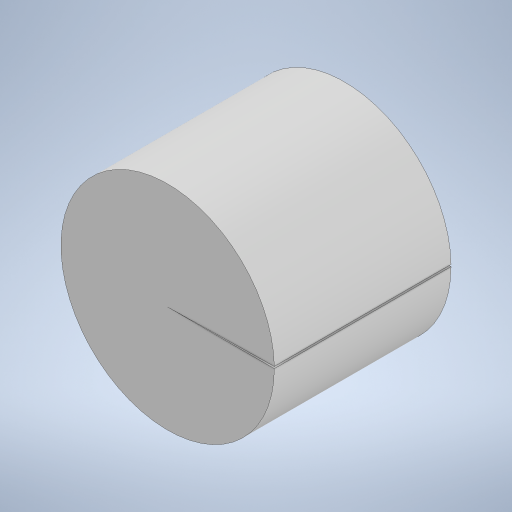
# Autodesk Inventor part: Espira_01_desarrollo
Saved by Autodesk Inventor 2024 (Build 280153000, 153)
## iProperties
Created: 2026-01-07
Part Number: Espira_01_desarrollo
Material: Generic
Document SubType Name: Modeling
Designer: eduso
Density: 1 g/cm^3
Appearance: Default
Author: eduso
Autodesk Inventor part; units mm, degrees
ref_plane "YZ Plane" through (0, 0, 0) normal (1, 0, 0) x (0, 1, 0)
ref_plane "XZ Plane" through (0, 0, 0) normal (0, 1, 0) x (-1, 0, 0)
ref_plane "XY Plane" through (0, 0, 0) normal (0, 0, 1) x (1, 0, 0)
sketch "Sketch1" plane through (0, 0, 0) normal (0, 0, 1) x (1, 0, 0)
  arc A0 (1.0919, 0.0191) -> (1.0921, 0) centre (0, 0) ccw
  arc A1 (3.6216, 0.0632) -> (3.6221, 0) centre (0, 0) ccw
  line L0 (0, 0) -> (3.6221, 0)
  line L1 (0, 0) -> (3.6216, 0.0632)
  dimension "d0" = 2.1841
  dimension "d1" = 7.2443
  dimension "d2" = 359
  constraints: 4 end point, 4 point on circle, 2 centre point, 2 coincident, 2 point on line, 1 horizontal
  measures "d0" diameter of A0
  measures "d1" diameter of A1
extrude "Extrusion1" add sketch "Sketch1" along normal blind 6
equation "\"d0\" = Rint2"
equation "\"d1\" = Rext2"
equation "\"d2\" = Ang"
equation "\"d3\" = Espesor"
equation "\"Dia_Int_Esp\" = 60.3"
equation "\"Espesor\" = 6"
equation "\"Num_Vueltas\" = 1"
equation "\"Dm\" = 0.5 * Dia_Int_Esp + 0.5 * Dia_Ext_Esp"
equation "\"Rext\" = 0.159155 * L"
equation "\"k_ext\" = 0"
equation "\"k_int\" = 0"
equation "\"Rext2\" = Rext + k_ext"
equation "\"Rint2\" = Rint - k_int"
equation "\"Ang\" = 359deg"
equation "\"Dia_Ext_Esp\" = 200"
equation "\"L\" = 45.517189"
equation "\"Rint\" = 2.184152"
body "Solid1"
